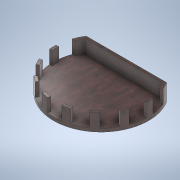
# Autodesk Inventor part: Nest-ver3-1111-2021
Saved by Autodesk Inventor 2021 (Build 250183000, 183)
## iProperties
Created: 2021-03-02
Part Number: Nest-ver3-1111-2021
Material: Generic
Document SubType Name: Modeling
Designer: CMurray
Density: 1 g/cm^3
Appearance: White Oak - Wild Berries
Author: CMurray
Autodesk Inventor part; units mm, degrees
ref_plane "YZ Plane" through (0, 0, 0) normal (1, 0, 0) x (0, 1, 0)
ref_plane "XZ Plane" through (0, 0, 0) normal (0, 1, 0) x (-1, 0, 0)
ref_plane "XY Plane" through (0, 0, 0) normal (0, 0, 1) x (1, 0, 0)
sketch "Sketch2" plane through (0, 0, 0) normal (0, 1, 0) x (-1, 0, 0)
  arc A0 (762, -479.9355) -> (-762, -479.9355) centre (0, 0) ccw
  line L0 (900.5455, 0) -> (762, 0)
  line L1 (762, -479.9355) -> (-762, -479.9355)
  dimension "d8" = 1524
  constraints: 4 end point, 3 point on circle, 1 centre point, 1 coincident, 1 horizontal
  measures "d8" distance of L1.start L1.end
extrude "Extrusion1" add sketch "Sketch2" along normal blind 63.5
sketch "Sketch9" plane through (0, 63.5, 0) normal (0, 1, 0) x (1, 0, 0)
  arc A0 (-762, 479.9355) -> (762, 479.9355) centre (0, 0) ccw
  line L0 (762, 479.9355) -> (-762, 479.9355) projected
  line L1 (-762, 479.9355) -> (762, 479.9355)
  constraints: 2 end point, 2 point on circle, 1 centre point, 1 coincident, 1 collinear
extrude "Extrusion10" add sketch "Sketch9" along normal blind 254
sketch "Sketch10" plane through (0, 317.5, 0) normal (0, 1, 0) x (1, 0, 0)
  arc A0 (-762, 479.9355) -> (762, 479.9355) centre (0, 0) ccw
  line L0 (762, 479.9355) -> (-762, 479.9355) projected
  line L1 (-762, 479.9355) -> (762, 479.9355)
  arc A1 (-733.4235, 429.1355) -> (733.4235, 429.1355) centre (0, 0) ccw
  line L2 (-733.4235, 429.1355) -> (733.4235, 429.1355)
  line L3 (-733.4235, 429.1355) -> (-791.7227, 429.1355)
  arc A2 (-762, 479.9355) -> (762, 479.9355) centre (0, 0) ccw projected
  line L4 (733.4235, 429.1355) -> (791.7227, 429.1355)
  line L5 (-794.2175, 302.1355) -> (-848.3491, 302.1355)
  line L6 (-848.381, 48.1355) -> (-899.0048, 48.1355)
  line L7 (-846.0779, -78.8645) -> (-891.7459, -78.8645)
  line L8 (-891.7459, -78.8645) -> (-897.0856, -78.8645)
  line L9 (-899.0048, 48.1355) -> (-899.2581, 48.1355)
  arc A3 (-762, 479.9355) -> (762, 479.9355) centre (0, 0) ccw projected
  line L10 (-784.9709, -325.4044) -> (-834.8069, -337.7567)
  line L11 (-784.9709, -325.4044) -> (-727.706, -438.7611)
  line L12 (-727.706, -438.7611) -> (-773.1686, -461.7276)
  line L13 (-565.5178, -634.2373) -> (-605.0317, -667.0223)
  line L14 (-565.5178, -634.2373) -> (-464.6758, -711.4378)
  line L15 (-464.6758, -711.4378) -> (-495.6377, -751.8812)
  line L16 (-233.6472, -816.9923) -> (-254.9841, -863.6928)
  line L17 (-109.2742, -842.69) -> (-119.5805, -892.5708)
  line L18 (144.6694, -837.3399) -> (145.7509, -888.6725)
  line L19 (267.8496, -806.4266) -> (280.2477, -855.8291)
  line L20 (494.2276, -691.2354) -> (517.5126, -736.9958)
  line L21 (591.7285, -609.8563) -> (625.6901, -650.5458)
  line L22 (745.5399, -407.7225) -> (786.3996, -438.8142)
  line L23 (797.9796, -292.0545) -> (844.3692, -313.0859)
  line L24 (848.6487, -43.1597) -> (899.5106, -43.1597)
  line L25 (845.6029, 83.8038) -> (896.5226, 85.0253)
  line L26 (783.0573, 329.9827) -> (832.8203, 342.6258)
  point P0 (624.3663, -648.9598)
  dimension "d44" = 50.8
  constraints: 52 end point, 6 horizontal, 6 point on circle, 2 perpendicular, 2 point on line, 1 centre point, 1 coincident, 39 other
extrude "Extrusion13" cut sketch "Sketch10" against normal blind 254 contours L5 A1 L6 L9 A0 | A0 L25 A1 L26 | L8 L7 A1 L10 A0 | A0 L23 A1 L24 | L12 A1 L13 A0 | A0 L21 A1 L22 | L15 A1 L16 A0 | A0 L19 A1 L20 | L17 A1 L18 A0
sketch "Sketch12" plane through (0, 317.5, 0) normal (0, 1, 0) x (1, 0, 0)
  arc A0 (899.5106, -43.1597) -> (896.5226, 85.0253) centre (0, 0) ccw projected
  arc A1 (-762, 479.9355) -> (762, 479.9355) centre (0, 0) ccw
  line L0 (762, 479.9355) -> (-762, 479.9355) projected
  line L1 (-762, 479.9355) -> (762, 479.9355)
  arc A2 (-733.4235, 429.1355) -> (733.4235, 429.1355) centre (0, 0) ccw
  line L2 (-733.4235, 429.1355) -> (733.4235, 429.1355)
  dimension "d73" = 50.8
  constraints: 5 point on circle, 4 end point, 2 centre point, 1 coincident, 1 collinear, 1 other
  measures "d73" radial gap between concentric circles of A1 A2
extrude "Extrusion14" cut sketch "Sketch12" against normal blind 254 contours L2 A2
body "Solid1"
